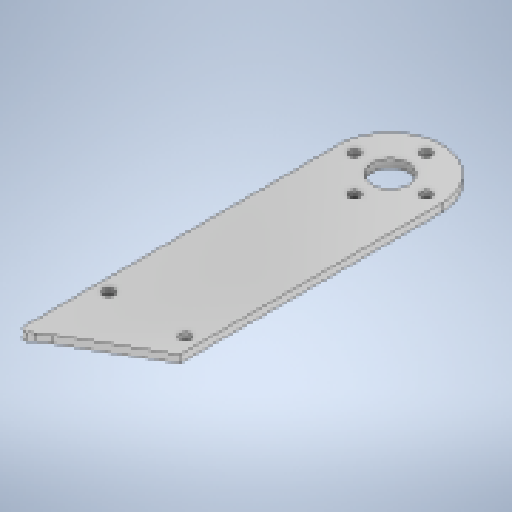
# Autodesk Inventor part: axis_8_10_connector_frame
Saved by Autodesk Inventor 2025.2 (Build 292293000, 293)
## iProperties
Created: 2025-05-04
Part Number: axis_8_10_connector_frame
Material: Aluminum 6061-AHC
Document SubType Name: Sheet Metal
Designer: User
Density: 2.7 g/cm^3
Sheet Metal Rule: Default_mm
Appearance: Aluminum - Dark
Author: User
Autodesk Inventor part; units mm, degrees
ref_plane "YZ Plane" through (0, 0, 0) normal (1, 0, 0) x (0, 1, 0)
ref_plane "XZ Plane" through (0, 0, 0) normal (0, 1, 0) x (-1, 0, 0)
ref_plane "XY Plane" through (0, 0, 0) normal (0, 0, 1) x (1, 0, 0)
sketch "Sketch1" plane through (0, 0, 0) normal (0, 1, 0) x (-1, 0, 0)
  line L0 (10, -35) -> (-10, -35)
  line L1 (-10, -35) -> (-10, 39.4211)
  line L2 (10, 39.4211) -> (10, -35)
  arc A0 (-10, 39.4211) -> (10, 39.4211) centre (0, 45.1) ccw
  point P0 (0, 0)
  dimension "d2" = 35
  dimension "d3" = 10
  dimension "d36" = 23
  dimension "d37" = 80.1
  dimension "d39" = 74.4211
  dimension "d40" = 20
  measures "d2" distance from line of L0 point (0, 0)
  measures "d3" distance from line of point (0, 0) L1
  measures "d36" diameter of A0
  measures "d37" distance from line of A0.centre L0
  measures "d39" distance of L2.start L0.start
  measures "d40" distance between parallel lines of L1 L2
extrude "Plate1" add sketch "Sketch1" along normal blind 1.5
sketch "Sketch3" plane through (0, 1.5, 0) normal (0, 1, 0) x (1, 0, 0)
  circle A0 centre (0, 25) radius 10
  circle A1 centre (0, -25) radius 10
  line L0 (-10, 35) -> (10, 35) projected
  line L1 (10, -44) -> (-10, -44) projected
  line L2 (-10, 35) -> (10, 35)
  line L3 (10, 35) -> (10, 25)
  line L4 (10, 25) -> (-10, 25)
  line L5 (-10, 25) -> (-10, 35)
  line L6 (10, -35) -> (-10, -35)
  line L7 (-10, -35) -> (-10, -25)
  line L8 (-10, -25) -> (10, -25)
  line L9 (10, -25) -> (10, -44)
  point P0 (0, 0)
  point P1 (-10, -39.4211)
  point P2 (10, -25)
  point P3 (0, -35)
  point P4 (-10, -35)
  point P5 (0, 35)
  point P6 (10, 35)
  dimension "d12" = 20
  dimension "d13" = 20
  dimension "d14" = 10
  dimension "d15" = 10
  dimension "d16" = 25
  dimension "d17" = 25
  dimension "d18" = 10
  constraints: 16 end point, 4 parallel, 2 horizontal, 2 perpendicular, 1 point on line, 7 other
  measures "d14" distance from line of L0 point (0, 25)
  measures "d16" distance of point (0, 0) point (0, 25)
  measures "d17" distance of point (0, 0) point (0, -25)
  measures "d18" distance of L2.end L3.end
extrude "Extrusion1" cut sketch "Sketch3" against normal blind 10 contours L5 L0 A0 | A0 L0 L3
sketch "Sketch4" plane through (0, 1.5, 0) normal (0, 1, 0) x (1, 0, 0)
  circle A0 centre (-7, 25) radius 0.8
  arc A1 (10, 25) -> (-10, 25) centre (0, 25) ccw projected
  circle A2 centre (0, 18) radius 0.8
  circle A3 centre (7, 25) radius 0.8
  circle A4 centre (0, 32) radius 0.8
  point P0 (0, 0)
  dimension "d21" = 0
  dimension "d22" = 7
  dimension "d23" = 1.6
  dimension "d26" = 360
  constraints: 4 centre point, 9 other
  measures "d21" vertical distance of A1.centre A0.centre
  measures "d22" distance of A1.centre A0.centre
  measures "d23" diameter of A0
hole "Hole2" at (0, 1.5, -32) at (7, 1.5, -25) at (0, 1.5, -18) at (-7, 1.5, -25) direction (0, -1, 0) diameter 2.1 depth 1.5
fillet "Fillet1" radius 1 2 edges at (-10, 0.75, 39.4211) (10, 0.75, 39.4211)
sketch "Sketch5" plane through (0, 1.5, 0) normal (0, 1, 0) x (1, 0, 0)
  arc A0 (10, 25) -> (-10, 25) centre (0, 25) ccw projected
  point P0 (0, 0)
hole "Hole3" at (0, 1.5, -25) direction (0, -1, 0) diameter 7.2 depth 1.5
sketch "Sketch8" plane through (0, 1.5, 0) normal (0, 1, 0) x (1, 0, 0)
  line L0 (19.8447, -20.3636) -> (-14.9774, -40.4682)
  arc A0 (8.28, -37.1193) -> (-8.28, -37.1193) centre (0, -45.1) ccw projected
  arc A1 (8.28, -37.1193) -> (10, -36.4253) centre (9, -36.4253) ccw projected
  line L1 (10, 25) -> (10, -36.4253) projected
  point P0 (0, 0)
  point P1 (10, -26.0474)
  point P2 (-5.75, -35.1407)
  dimension "d63" = 60
  constraints: 2 end point, 1 tangent
  measures "d63" angle of L0 L1
extrude "Extrusion2" cut sketch "Sketch8" against normal blind 1.5
equation "\"d33\" = Thickness"
equation "\"d47\" = Thickness"
equation "\"d4\" = Thickness"
equation "\"BendReliefWidth\" = Thickness"
equation "\"BendReliefDepth\" = 0.5 * Thickness"
equation "\"CornerReliefSize\" = 4 * Thickness"
equation "\"MinimumRemnant\" = 2 * Thickness"
equation "\"TransitionRadius\" = BendRadius"
equation "\"JacobiRadiusSize\" = BendRadius"
equation "\"GapSize\" = Thickness"
equation "\"Thickness\" = 1.5"
equation "\"BendRadius\" = 0.31"
body "Solid1"
